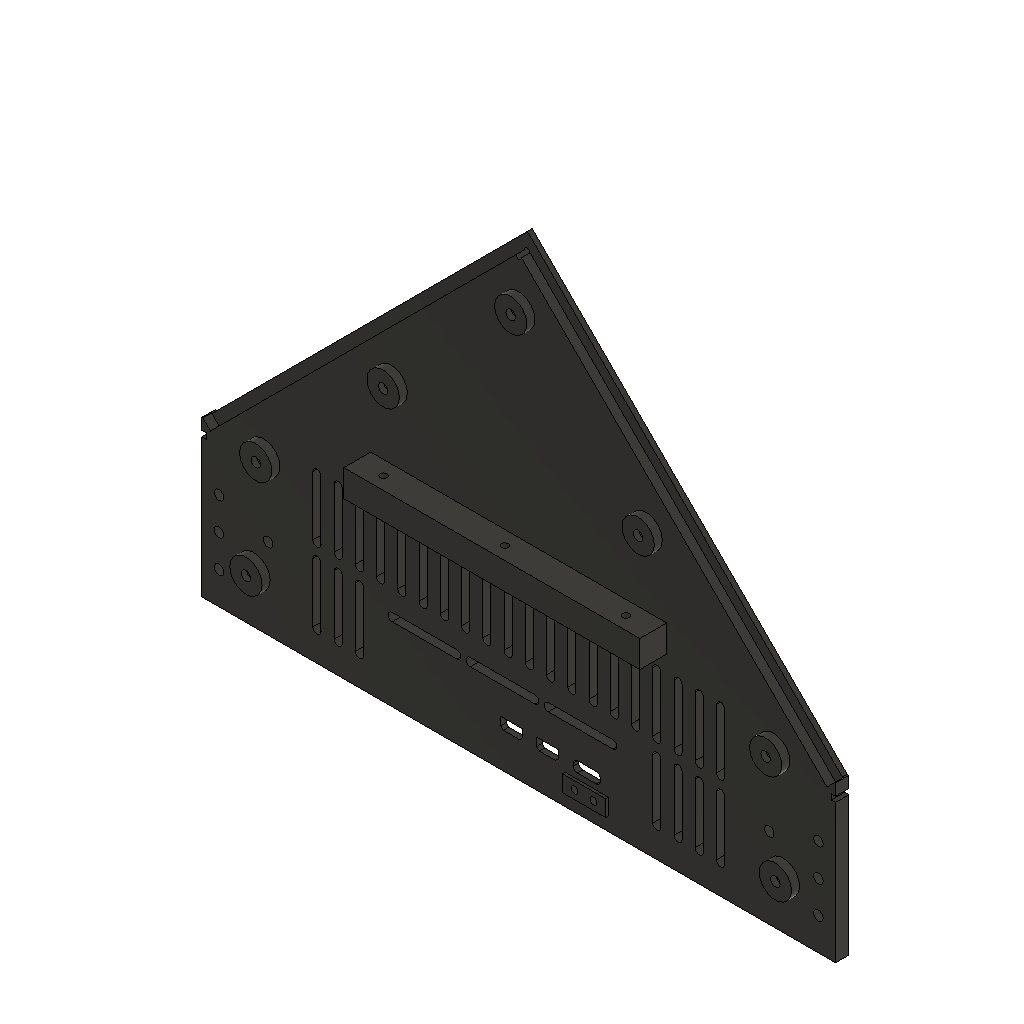
back (Autodesk Fusion 360 design; units mm, degrees)
Autodesk Fusion 360 part; units mm, degrees
sketch "Skizze1" plane through (0, 0, 0) normal (0, 1, 0) x (1, 0, 0)
  line L0 (-3.3486, -96.1672) -> (-1.6743, -99.0672)
  circle A0 centre (0, -113.552) radius 1
  line L1 (-1.6743, -99.0672) -> (1.6743, -99.0672)
  circle A1 centre (47.3762, -48.7911) radius 1.75
  circle A2 centre (47.3762, -48.7911) radius 6
  line L2 (116.137, 3.4146) -> (118.137, 3.4146)
  line L3 (96.4266, 1.4851) -> (98.1009, -1.4149)
  line L4 (93.078, -4.3149) -> (91.4037, -1.4149)
  line L5 (50.7248, -48.7911) -> (49.0505, -51.6911)
  line L6 (118.137, 3.4146) -> (118.137, 1.4146)
  line L7 (93.078, 1.4851) -> (96.4266, 1.4851)
  line L8 (1.6743, -99.0672) -> (3.3486, -96.1672)
  circle A3 centre (0, -96.1672) radius 1.75
  line L9 (114.552, 0) -> (117.3804, -2.8284)
  circle A4 centre (94.7523, -1.4149) radius 1.75
  line L10 (3.3486, -96.1672) -> (1.6743, -93.2672)
  circle A5 centre (94.7523, -1.4149) radius 6
  line L11 (0, -120.2089) -> (117.3804, -2.8284)
  line L12 (45.7018, -45.8911) -> (49.0505, -45.8911)
  circle A6 centre (-111.38, 31) radius 1.75
  line L13 (-49.0505, -45.8911) -> (-50.7248, -48.7911)
  line L14 (-45.7018, -45.8911) -> (-49.0505, -45.8911)
  line L15 (-100.0543, 34.1) -> (-96.7057, 34.1)
  circle A7 centre (-111.38, 43) radius 1.75
  line L16 (-118.137, -2.8284) -> (-118.137, 55)
  line L17 (-100.0543, 39.9) -> (-101.7286, 37)
  line L18 (-120.0068, 23.8396) -> (4.4419, -100.6092) construction
  circle A8 centre (-94.7523, -1.4149) radius 1.75
  line L19 (-14.6701, -110.8373) -> (106.0816, 9.9144) construction
  line L20 (-111.38, -4.6505) -> (-111.38, 58.1997) construction
  circle A9 centre (-98.38, 37) radius 6
  line L21 (-96.7057, 34.1) -> (-95.0314, 37)
  circle A10 centre (-94.7523, -1.4149) radius 6
  line L22 (-52.4459, 0) -> (345.6761, 0) construction
  line L23 (-118.137, 55) -> (118.137, 55)
  line L24 (-116.137, 1.4146) -> (-116.137, 3.4146)
  line L25 (-117.3804, -2.8284) -> (-118.137, -2.8284)
  line L26 (-114.552, 0) -> (0, -114.552)
  line L27 (-95.0314, 37) -> (-96.7057, 39.9)
  line L28 (-118.137, 3.4146) -> (-118.137, 1.4146)
  line L29 (-96.7057, 39.9) -> (-100.0543, 39.9)
  line L30 (-96.4266, 1.4851) -> (-98.1009, -1.4149)
  line L31 (-116.137, 3.4146) -> (-118.137, 3.4146)
  line L32 (-93.078, -4.3149) -> (-91.4037, -1.4149)
  line L33 (-91.4037, -1.4149) -> (-93.078, 1.4851)
  line L34 (-118.137, 1.4146) -> (-116.137, 1.4146)
  circle A11 centre (-93.137, 25) radius 1.75
  line L35 (-98.38, 29.5228) -> (-98.38, 65.4203) construction
  line L36 (-93.137, 11.8531) -> (-93.137, 59.4737) construction
  line L37 (-98.1009, -1.4149) -> (-96.4266, -4.3149)
  line L38 (-93.078, 1.4851) -> (-96.4266, 1.4851)
  circle A12 centre (-98.38, 37) radius 1.75
  line L39 (-96.4266, -4.3149) -> (-93.078, -4.3149)
  line L40 (-114.552, 0) -> (-117.3804, -2.8284)
  circle A13 centre (-111.38, 19) radius 1.75
  line L41 (-101.7286, 37) -> (-100.0543, 34.1)
  line L42 (91.4037, -1.4149) -> (93.078, 1.4851)
  circle A14 centre (-47.3762, -48.7911) radius 6
  line L43 (-44.0275, -48.7911) -> (-45.7018, -45.8911)
  line L44 (-45.7018, -51.6911) -> (-44.0275, -48.7911)
  line L45 (-49.0505, -51.6911) -> (-45.7018, -51.6911)
  circle A15 centre (-47.3762, -48.7911) radius 1.75
  line L46 (118.137, -2.8284) -> (118.137, 55)
  line L47 (100.0543, 34.1) -> (96.7057, 34.1)
  line L48 (-117.3804, -2.8284) -> (0, -120.2089)
  line L49 (96.7057, 39.9) -> (100.0543, 39.9)
  line L50 (100.0543, 39.9) -> (101.7286, 37)
  line L51 (0, -220.0498) -> (0, 135.0469) construction
  line L52 (111.38, -16.7918) -> (111.38, 73.2082) construction
  line L53 (-0.5511, 92.7863) -> (31.9162, 125.2536) construction
  circle A16 centre (111.38, 19) radius 1.75
  circle A17 centre (111.38, 43) radius 1.75
  line L54 (95.0314, 37) -> (96.7057, 39.9)
  circle A18 centre (111.38, 31) radius 1.75
  line L55 (-50.7248, -48.7911) -> (-49.0505, -51.6911)
  line L56 (116.137, 1.4146) -> (116.137, 3.4146)
  line L57 (101.7286, 37) -> (100.0543, 34.1)
  circle A19 centre (98.38, 37) radius 6
  circle A20 centre (93.137, 25) radius 1.75
  circle A21 centre (98.38, 37) radius 1.75
  line L58 (45.7018, -51.6911) -> (44.0275, -48.7911)
  line L59 (1.6743, -93.2672) -> (-1.6743, -93.2672)
  line L60 (118.137, 1.4146) -> (116.137, 1.4146)
  line L61 (96.7057, 34.1) -> (95.0314, 37)
  line L62 (98.1009, -1.4149) -> (96.4266, -4.3149)
  line L63 (49.0505, -45.8911) -> (50.7248, -48.7911)
  line L64 (-1.6743, -93.2672) -> (-3.3486, -96.1672)
  circle A22 centre (0, -96.1672) radius 6
  line L65 (44.0275, -48.7911) -> (45.7018, -45.8911)
  line L66 (49.0505, -51.6911) -> (45.7018, -51.6911)
  line L67 (96.4266, -4.3149) -> (93.078, -4.3149)
  line L68 (117.3804, -2.8284) -> (118.137, -2.8284)
  line L69 (0, -114.552) -> (114.552, 0)
  line L70 (34.8, 35.9) -> (-10.8, 35.9)
  line L71 (-10.8, 35.9) -> (-10.8, 43.9)
  line L72 (-10.8, 43.9) -> (34.8, 43.9)
  line L73 (34.8, 43.9) -> (34.8, 35.9)
  line L74 (37, 50) -> (-32, 50) construction
  line L75 (51.4459, 39.9) -> (-23, 39.9) construction
  line L76 (10.7, 28) -> (10.7, 48) construction
  line L77 (25.3, 21.2933) -> (25.3, 58) construction
  line L78 (-2.7, 28) -> (-2.7, 48) construction
  line L79 (21.8, 41.9) -> (28.8, 41.9)
  line L80 (30.3, 40.4) -> (30.3, 39.4)
  line L81 (28.8, 37.9) -> (21.8, 37.9)
  line L82 (20.3, 39.4) -> (20.3, 40.4)
  line L83 (20.3, 41.9) -> (30.3, 37.9) construction
  line L84 (30.3, 41.9) -> (20.3, 37.9) construction
  line L85 (7.7, 41.9) -> (13.7, 41.9)
  line L86 (14.7, 40.9) -> (14.7, 37.9)
  line L87 (14.7, 37.9) -> (6.7, 37.9)
  line L88 (6.7, 37.9) -> (6.7, 40.9)
  line L89 (6.7, 41.9) -> (14.7, 37.9) construction
  line L90 (14.7, 41.9) -> (6.7, 37.9) construction
  line L91 (-5.7, 41.9) -> (0.3, 41.9)
  line L92 (1.3, 40.9) -> (1.3, 37.9)
  line L93 (1.3, 37.9) -> (-6.7, 37.9)
  line L94 (-6.7, 37.9) -> (-6.7, 40.9)
  line L95 (-6.7, 41.9) -> (1.3, 37.9) construction
  line L96 (1.3, 41.9) -> (-6.7, 37.9) construction
  arc A23 (28.8, 37.9) -> (30.3, 39.4) centre (28.8, 39.4) ccw
  arc A24 (20.3, 39.4) -> (21.8, 37.9) centre (21.8, 39.4) ccw
  arc A25 (21.8, 41.9) -> (20.3, 40.4) centre (21.8, 40.4) ccw
  arc A26 (30.3, 40.4) -> (28.8, 41.9) centre (28.8, 40.4) ccw
  line L97 (1.3, 40.9) -> (0.3, 41.9)
  line L98 (-5.7, 41.9) -> (-6.7, 40.9)
  line L99 (7.7, 41.9) -> (6.7, 40.9)
  line L100 (13.7, 41.9) -> (14.7, 40.9)
  line L101 (38, 46.9) -> (16.3042, 46.9) construction
  line L102 (33.3, 43.9) -> (33.3, 50)
  line L103 (17.3, 43.9) -> (17.3, 50)
  line L104 (33.3, 50) -> (17.3, 50)
  line L105 (28.8, 44.4473) -> (28.8, 49) construction
  line L106 (21.8, 44.3848) -> (21.8, 49.4152) construction
  circle A27 centre (28.8, 46.9) radius 1.25
  circle A28 centre (21.8, 46.9) radius 1.25
  line L107 (27.5298, 49.1) -> (26.2597, 46.9)
  line L108 (26.2597, 46.9) -> (27.5298, 44.7)
  line L109 (27.5298, 44.7) -> (30.0702, 44.7)
  line L110 (30.0702, 44.7) -> (31.3403, 46.9)
  line L111 (31.3403, 46.9) -> (30.0702, 49.1)
  line L112 (30.0702, 49.1) -> (27.5298, 49.1)
  line L113 (20.5298, 49.1) -> (19.2597, 46.9)
  line L114 (19.2597, 46.9) -> (20.5298, 44.7)
  line L115 (20.5298, 44.7) -> (23.0702, 44.7)
  line L116 (23.0702, 44.7) -> (24.3403, 46.9)
  line L117 (24.3403, 46.9) -> (23.0702, 49.1)
  line L118 (23.0702, 49.1) -> (20.5298, 49.1)
  line L119 (130, -23) -> (-128.9642, -23) construction
  line L120 (-55, -13) -> (55, -13)
  line L121 (55, -13) -> (55, -23)
  line L122 (55, -23) -> (-55, -23)
  line L123 (-55, -23) -> (-55, -13)
  line L124 (-55, -13) -> (55, -23) construction
  line L125 (55, -13) -> (-55, -23) construction
  line L126 (65.5233, 43.1) -> (-51.9095, 43.1) construction
  line L127 (67.4251, 23.1) -> (-80, 23.1) construction
  line L128 (73.5779, 26.1) -> (-77.6362, 26.1) construction
  line L129 (36.5, 19) -> (36.5, 58) construction
  line L130 (-48.5, 15) -> (-48.5, 73) construction
  line L131 (-47, 27.6) -> (-23, 27.6)
  line L132 (-23, 27.6) -> (-23, 24.6) construction
  line L133 (-23, 24.6) -> (-47, 24.6)
  line L134 (-47, 24.6) -> (-47, 27.6) construction
  line L135 (-47, 27.6) -> (-23, 24.6) construction
  line L136 (-23, 27.6) -> (-47, 24.6) construction
  line L137 (-18, 27.6) -> (6, 27.6)
  line L138 (6, 27.6) -> (6, 24.6) construction
  line L139 (6, 24.6) -> (-18, 24.6)
  line L140 (-18, 24.6) -> (-18, 27.6) construction
  line L141 (-18, 27.6) -> (6, 24.6) construction
  line L142 (6, 27.6) -> (-18, 24.6) construction
  line L143 (11, 27.6) -> (35, 27.6)
  line L144 (35, 27.6) -> (35, 24.6) construction
  line L145 (35, 24.6) -> (11, 24.6)
  line L146 (11, 24.6) -> (11, 27.6) construction
  line L147 (11, 27.6) -> (35, 24.6) construction
  line L148 (35, 27.6) -> (11, 24.6) construction
  arc A29 (-47, 27.6) -> (-47, 24.6) centre (-47, 26.1) ccw
  arc A30 (-23, 24.6) -> (-23, 27.6) centre (-23, 26.1) ccw
  arc A31 (-18, 27.6) -> (-18, 24.6) centre (-18, 26.1) ccw
  arc A32 (6, 24.6) -> (6, 27.6) centre (6, 26.1) ccw
  arc A33 (11.4382, 27.5346) -> (11, 24.6) centre (11, 26.1) ccw
  arc A34 (35, 24.6) -> (35, 27.6) centre (35, 26.1) ccw
  line L149 (84.4109, 5) -> (-85.7418, 5) construction
  line L150 (73.5, 16) -> (76.5, 16) construction
  line L151 (76.5, 16) -> (76.5, -6)
  line L152 (76.5, -6) -> (73.5, -6) construction
  line L153 (73.5, -6) -> (73.5, 16)
  line L154 (73.5, 16) -> (76.5, -6) construction
  line L155 (76.5, 16) -> (73.5, -6) construction
  arc A35 (73.5, -6) -> (76.5, -6) centre (75, -6) ccw
  arc A36 (76.5, 16) -> (73.5, 16) centre (75, 16) ccw
  line L156 (65.6053, -6) -> (65.6053, 16)
  arc A37 (65.6053, -6) -> (68.6053, -6) centre (67.1053, -6) ccw
  line L157 (68.6053, 16) -> (68.6053, -6)
  arc A38 (68.6053, 16) -> (65.6053, 16) centre (67.1053, 16) ccw
  line L158 (57.7105, -6) -> (57.7105, 16)
  arc A39 (57.7105, -6) -> (60.7105, -6) centre (59.2105, -6) ccw
  line L159 (60.7105, 16) -> (60.7105, -6)
  arc A40 (60.7105, 16) -> (57.7105, 16) centre (59.2105, 16) ccw
  line L160 (49.8158, -6) -> (49.8158, 16)
  arc A41 (49.8158, -6) -> (52.8158, -6) centre (51.3158, -6) ccw
  line L161 (52.8158, 16) -> (52.8158, -6)
  arc A42 (52.8158, 16) -> (49.8158, 16) centre (51.3158, 16) ccw
  line L162 (41.9211, -6) -> (41.9211, 16)
  arc A43 (41.9211, -6) -> (44.9211, -6) centre (43.4211, -6) ccw
  line L163 (44.9211, 16) -> (44.9211, -6)
  arc A44 (44.9211, 16) -> (41.9211, 16) centre (43.4211, 16) ccw
  line L164 (34.0263, -6) -> (34.0263, 16)
  arc A45 (34.0263, -6) -> (37.0263, -6) centre (35.5263, -6) ccw
  line L165 (37.0263, 16) -> (37.0263, -6)
  arc A46 (37.0263, 16) -> (34.0263, 16) centre (35.5263, 16) ccw
  line L166 (26.1316, -6) -> (26.1316, 16)
  arc A47 (26.1316, -6) -> (29.1316, -6) centre (27.6316, -6) ccw
  line L167 (29.1316, 16) -> (29.1316, -6)
  arc A48 (29.1316, 16) -> (26.1316, 16) centre (27.6316, 16) ccw
  line L168 (18.2368, -6) -> (18.2368, 16)
  arc A49 (18.2368, -6) -> (21.2368, -6) centre (19.7368, -6) ccw
  line L169 (21.2368, 16) -> (21.2368, -6)
  arc A50 (21.2368, 16) -> (18.2368, 16) centre (19.7368, 16) ccw
  line L170 (10.3421, -6) -> (10.3421, 16)
  arc A51 (10.3421, -6) -> (13.3421, -6) centre (11.8421, -6) ccw
  line L171 (13.3421, 16) -> (13.3421, -6)
  arc A52 (13.3421, 16) -> (10.3421, 16) centre (11.8421, 16) ccw
  line L172 (2.4474, -6) -> (2.4474, 16)
  arc A53 (2.4474, -6) -> (5.4474, -6) centre (3.9474, -6) ccw
  line L173 (5.4474, 16) -> (5.4474, -6)
  arc A54 (5.4474, 16) -> (2.4474, 16) centre (3.9474, 16) ccw
  line L174 (-5.4474, -6) -> (-5.4474, 16)
  arc A55 (-5.4474, -6) -> (-2.4474, -6) centre (-3.9474, -6) ccw
  line L175 (-2.4474, 16) -> (-2.4474, -6)
  arc A56 (-2.4474, 16) -> (-5.4474, 16) centre (-3.9474, 16) ccw
  line L176 (-13.3421, -6) -> (-13.3421, 16)
  arc A57 (-13.3421, -6) -> (-10.3421, -6) centre (-11.8421, -6) ccw
  line L177 (-10.3421, 16) -> (-10.3421, -6)
  arc A58 (-10.3421, 16) -> (-13.3421, 16) centre (-11.8421, 16) ccw
  line L178 (-21.2368, -6) -> (-21.2368, 16)
  arc A59 (-21.2368, -6) -> (-18.2368, -6) centre (-19.7368, -6) ccw
  line L179 (-18.2368, 16) -> (-18.2368, -6)
  arc A60 (-18.2368, 16) -> (-21.2368, 16) centre (-19.7368, 16) ccw
  line L180 (-29.1316, -6) -> (-29.1316, 16)
  arc A61 (-29.1316, -6) -> (-26.1316, -6) centre (-27.6316, -6) ccw
  line L181 (-26.1316, 16) -> (-26.1316, -6)
  arc A62 (-26.1316, 16) -> (-29.1316, 16) centre (-27.6316, 16) ccw
  line L182 (-37.0263, -6) -> (-37.0263, 16)
  arc A63 (-37.0263, -6) -> (-34.0263, -6) centre (-35.5263, -6) ccw
  line L183 (-34.0263, 16) -> (-34.0263, -6)
  arc A64 (-34.0263, 16) -> (-37.0263, 16) centre (-35.5263, 16) ccw
  line L184 (-44.9211, -6) -> (-44.9211, 16)
  arc A65 (-44.9211, -6) -> (-41.9211, -6) centre (-43.4211, -6) ccw
  line L185 (-41.9211, 16) -> (-41.9211, -6)
  arc A66 (-41.9211, 16) -> (-44.9211, 16) centre (-43.4211, 16) ccw
  line L186 (-52.8158, -6) -> (-52.8158, 16)
  arc A67 (-52.8158, -6) -> (-49.8158, -6) centre (-51.3158, -6) ccw
  line L187 (-49.8158, 16) -> (-49.8158, -6)
  arc A68 (-49.8158, 16) -> (-52.8158, 16) centre (-51.3158, 16) ccw
  line L188 (-60.7105, -6) -> (-60.7105, 16)
  arc A69 (-60.7105, -6) -> (-57.7105, -6) centre (-59.2105, -6) ccw
  line L189 (-57.7105, 16) -> (-57.7105, -6)
  arc A70 (-57.7105, 16) -> (-60.7105, 16) centre (-59.2105, 16) ccw
  line L190 (-68.6053, -6) -> (-68.6053, 16)
  arc A71 (-68.6053, -6) -> (-65.6053, -6) centre (-67.1053, -6) ccw
  line L191 (-65.6053, 16) -> (-65.6053, -6)
  arc A72 (-65.6053, 16) -> (-68.6053, 16) centre (-67.1053, 16) ccw
  line L192 (-76.5, -6) -> (-76.5, 16)
  arc A73 (-76.5, -6) -> (-73.5, -6) centre (-75, -6) ccw
  line L193 (-73.5, 16) -> (-73.5, -6)
  arc A74 (-73.5, 16) -> (-76.5, 16) centre (-75, 16) ccw
  line L194 (86.8847, 33) -> (-89.6414, 33) construction
  line L195 (73.5, 44) -> (76.5, 44) construction
  line L196 (76.5, 44) -> (76.5, 22)
  line L197 (76.5, 22) -> (73.5, 22) construction
  line L198 (73.5, 22) -> (73.5, 44)
  line L199 (73.5, 44) -> (76.5, 22) construction
  line L200 (76.5, 44) -> (73.5, 22) construction
  arc A75 (73.5, 22) -> (76.5, 22) centre (75, 22) ccw
  arc A76 (76.5, 44) -> (73.5, 44) centre (75, 44) ccw
  line L201 (65.605, 22) -> (65.605, 44)
  arc A77 (65.605, 22) -> (68.605, 22) centre (67.105, 22) ccw
  line L202 (68.605, 44) -> (68.605, 22)
  arc A78 (68.605, 44) -> (65.605, 44) centre (67.105, 44) ccw
  line L203 (57.71, 22) -> (57.71, 44)
  arc A79 (57.71, 22) -> (60.71, 22) centre (59.21, 22) ccw
  line L204 (60.71, 44) -> (60.71, 22)
  arc A80 (60.71, 44) -> (57.71, 44) centre (59.21, 44) ccw
  line L205 (49.815, 22) -> (49.815, 44)
  arc A81 (49.815, 22) -> (52.815, 22) centre (51.315, 22) ccw
  line L206 (52.815, 44) -> (52.815, 22)
  arc A82 (52.815, 44) -> (49.815, 44) centre (51.315, 44) ccw
  line L207 (-76.5, 44) -> (-73.5, 44) construction
  line L208 (-73.5, 44) -> (-73.5, 22)
  line L209 (-73.5, 22) -> (-76.5, 22) construction
  line L210 (-76.5, 22) -> (-76.5, 44)
  line L211 (-76.5, 44) -> (-73.5, 22) construction
  line L212 (-73.5, 44) -> (-76.5, 22) construction
  arc A83 (-73.5, 22.0002) -> (-73.5, 22) centre (-72.7991, 22) ccw
  arc A84 (-73.5, 44) -> (-76.5, 44) centre (-75, 44) ccw
  arc A85 (-76.5, 22) -> (-73.5, 22.0002) centre (-75, 22) ccw
  line L213 (-68.605, 22) -> (-68.605, 44)
  arc A86 (-68.605, 22) -> (-65.605, 22.0002) centre (-67.105, 22) ccw
  line L214 (-65.605, 44) -> (-65.605, 22)
  arc A87 (-65.605, 44) -> (-68.605, 44) centre (-67.105, 44) ccw
  line L215 (-60.71, 22) -> (-60.71, 44)
  arc A88 (-60.71, 22) -> (-57.71, 22.0002) centre (-59.21, 22) ccw
  line L216 (-57.71, 44) -> (-57.71, 22)
  arc A89 (-57.71, 44) -> (-60.71, 44) centre (-59.21, 44) ccw
  point P0 (114.552, 0)
  point P1 (-114.552, 0)
  point P2 (-94.7523, -1.4149)
  point P3 (-98.38, 37)
  point P4 (0, -96.1672)
  point P5 (0, -16.1)
  point P6 (0, 46.6)
  point P7 (-47.3762, -48.7911)
  point P8 (25.3, 39.9)
  point P9 (10.7, 39.9)
  point P10 (-2.7, 39.9)
  point P11 (28.8, 46.9)
  point P12 (21.8, 46.9)
  point P13 (0, -18)
  point P14 (-35, 26.1)
  point P15 (-6, 26.1)
  point P16 (23, 26.1)
  point P17 (75, 5)
  point P18 (75, 33)
  point P19 (75, 22)
  point P20 (-75, 33)
  dimension "d1" = 55
  dimension "d2" = 45
  dimension "d3" = 4
  dimension "d4" = 4
  dimension "d5" = 12
  dimension "d6" = 12
  dimension "d7" = 12
  dimension "d8" = 3.5
  dimension "d9" = 3.5
  dimension "d10" = 3.5
  dimension "d11" = 12
  dimension "d12" = 12
  dimension "d13" = 12
  dimension "d14" = 3.5
  dimension "d15" = 3.5
  dimension "d16" = 3.5
  dimension "d17" = 18
  dimension "d18" = 12
  dimension "d19" = 3.5
  dimension "d20" = 5.8
  dimension "d21" = 3.5
  dimension "d22" = 30
  dimension "d23" = 13
  dimension "d25" = 13
  dimension "d26" = 3.5
  dimension "d27" = 12
  dimension "d28" = 5.8
  dimension "d29" = 12
  dimension "d30" = 3.5
  dimension "d31" = 5.8
  dimension "d33" = 12
  dimension "d34" = 3.5
  dimension "d35" = 5.8
  dimension "d42" = 118.137
  dimension "d43" = 6.757
  dimension "d44" = 19.757
  dimension "d45" = 25
  dimension "d46" = 3.585
  dimension "d47" = 118.137
  dimension "d48" = 6.757
  dimension "d49" = 3.585
  dimension "d50" = 4.243
  dimension "d51" = 2
  dimension "d52" = 2
  dimension "d53" = 2
  dimension "d54" = 11.1
  dimension "d55" = 5
  dimension "d56" = 34.8
  dimension "d57" = 10.8
  dimension "d58" = 4
  dimension "d59" = 4
  dimension "d60" = 21.5
  dimension "d61" = 14.6
  dimension "d62" = 13.4
  dimension "d63" = 4
  dimension "d64" = 10
  dimension "d65" = 1.5
  dimension "d66" = 4
  dimension "d67" = 8
  dimension "d68" = 4
  dimension "d69" = 8
  dimension "d70" = 1
  dimension "d71" = 1
  dimension "d72" = 1
  dimension "d73" = 1
  dimension "d74" = 1
  dimension "d75" = 1
  dimension "d76" = 1
  dimension "d77" = 1
  dimension "d78" = 7
  dimension "d79" = 8
  dimension "d80" = 8
  dimension "d81" = 3.5
  dimension "d82" = 3.5
  dimension "d83" = 2.5
  dimension "d84" = 2.5
  dimension "d85" = 4.4
  dimension "d86" = 4.4
  dimension "d91" = 67
  dimension "d92" = 67
  dimension "d113" = 78
  dimension "d114" = 10
  dimension "d115" = 110
  dimension "d133" = 3.2
  dimension "d134" = 20
  dimension "d135" = 3
  dimension "d136" = 11.2
  dimension "d137" = 85
  dimension "d138" = 3
  dimension "d139" = 3
  dimension "d140" = 3
  dimension "d141" = 24
  dimension "d142" = 24
  dimension "d143" = 42.5
  dimension "d144" = 24
  dimension "d145" = 29
  dimension "d146" = 29
  dimension "d147" = 3
  dimension "d148" = 22
  dimension "d151" = -150
  dimension "d152" = 0
  dimension "d153" = 75
  dimension "d154" = 50
  dimension "d155" = 3
  dimension "d156" = 22
  dimension "d158" = 75
  dimension "d159" = 22
  dimension "d162" = -23.685
  dimension "d163" = 0
  dimension "d164" = 3
  dimension "d165" = 22
  dimension "d166" = 75
  dimension "d169" = 15.79
  dimension "d170" = 0
  constraint horizontal L22
  constraint coincident origin L51
  constraint coincident origin L22
  constraint horizontal L23
  constraint coincident P1 L22
  constraint coincident P0 L22
  constraint coincident P1 L26.start
  constraint coincident L26.end L51
  constraint coincident P0 L9.start
  constraint perpendicular L26 L40
  constraint perpendicular L9 L69
  constraint horizontal L68
  constraint perpendicular L20 L23
  constraint perpendicular L23 L52
  constraint coincident A17.centre L52
  constraint coincident A18.centre L52
  constraint coincident A16.centre L52
  constraint coincident A7.centre L20
  constraint coincident A6.centre L20
  constraint coincident A13.centre L20
  constraint perpendicular L23 L35
  constraint coincident P3 L35
  constraint concentric A9 A12
  constraint coincident P3 A9.centre
  constraint horizontal L29
  constraint perpendicular L23 L36
  constraint coincident A11.centre L36
  constraint parallel L18 L26
  constraint parallel L19 L69
  constraint coincident P4 L51
  constraint coincident P4 L18
  constraint concentric A3 A22
  constraint coincident P4 A3.centre
  constraint horizontal L1
  constraint coincident P7 L18
  constraint concentric A14 A15
  constraint coincident P7 A14.centre
  constraint horizontal L14
  constraint perpendicular L18 L53
  constraint coincident P2 L18
  constraint coincident P2 L53
  constraint concentric A8 A10
  constraint coincident P2 A8.centre
  constraint horizontal L38
  constraint symmetric A9 L51 A19
  constraint symmetric A12 L51 A21
  constraint symmetric L17.start L49.end L51
  constraint symmetric L17.end L50.end L51
  constraint symmetric L15.start L47.start L51
  constraint symmetric L15.end L47.end L51
  constraint symmetric L54.start L21.end L51
  constraint symmetric L49.start L27.end L51
  constraint symmetric A11 L51 A20
  constraint symmetric A1 A15 L51
  constraint symmetric A2 A14 L51
  constraint symmetric L12.end L13.start L51
  constraint symmetric L13.end L5.start L51
  constraint symmetric L5.end L45.start L51
  constraint symmetric L58.start L44.start L51
  constraint symmetric L58.end L43.start L51
  constraint symmetric L12.start L14.start L51
  constraint symmetric A4 A8 L51
  constraint symmetric A5 A10 L51
  constraint symmetric L3.start L30.start L51
  constraint symmetric L3.end L30.end L51
  constraint symmetric L37.end L62.end L51
  constraint symmetric L32.start L4.start L51
  constraint symmetric L32.end L4.end L51
  constraint symmetric L33.end L7.start L51
  constraint coincident P6 L51
  constraint coincident P5 L51
  constraint coincident L11.start L51
  constraint parallel L26 L48
  constraint coincident L16.end L23
  constraint perpendicular L16 L23
  constraint coincident L25.end L16
  constraint coincident L16.end L23.start
  constraint coincident L46.start L68
  constraint coincident L46.end L23
  constraint perpendicular L23 L46
  constraint coincident L23.end L46.end
  constraint coincident L46.start L68.end
  constraint horizontal L34
  constraint vertical L24
  constraint horizontal L31
  constraint vertical L28
  constraint coincident L28.end L16
  constraint symmetric L28.end L6.end L51
  constraint symmetric L24.start L56.start L51
  constraint symmetric L24.end L2.start L51
  constraint symmetric L28.start L2.end L51
  constraint coincident A0.centre L51
  constraint coincident L26.end A0
  constraint horizontal L70
  constraint vertical L71
  constraint horizontal L72
  constraint vertical L73
  constraint perpendicular L71 L74
  constraint perpendicular L51 L75
  constraint perpendicular L72 L76
  constraint perpendicular L72 L77
  constraint perpendicular L72 L78
  constraint horizontal L79
  constraint perpendicular L79 L80
  constraint parallel L79 L81
  constraint parallel L80 L82
  constraint coincident L83 P8
  constraint coincident L84 P8
  constraint coincident L77 P8
  constraint coincident L75 P8
  constraint horizontal L85
  constraint perpendicular L85 L86
  constraint parallel L85 L87
  constraint parallel L86 L88
  constraint coincident L89 P9
  constraint coincident L90 P9
  constraint coincident L75 P9
  constraint coincident L76 P9
  constraint horizontal L91
  constraint perpendicular L91 L92
  constraint parallel L91 L93
  constraint parallel L92 L94
  constraint coincident L95 P10
  constraint coincident L96 P10
  constraint coincident L78 P10
  constraint coincident L75 P10
  constraint coincident L83.end L81
  constraint coincident L83.end L80
  constraint tangent L81 A23
  constraint tangent L80 A23
  constraint coincident L84.end L81
  constraint coincident L84.end L82
  constraint tangent L81 A24
  constraint tangent L82 A24
  constraint equal A23 A24
  constraint coincident L83.start L82
  constraint coincident L83.start L79
  constraint tangent L82 A25
  constraint tangent L79 A25
  constraint equal A23 A25
  constraint coincident L84.start L79
  constraint coincident L84.start L80
  constraint tangent L79 A26
  constraint tangent L80 A26
  constraint equal A23 A26
  constraint coincident L96.start L92
  constraint coincident L96.start L91
  constraint coincident L95.start L91
  constraint coincident L95.start L94
  constraint coincident L89.start L85
  constraint coincident L89.start L88
  constraint coincident L90.start L85
  constraint coincident L90.start L86
  constraint perpendicular L77 L101
  constraint coincident L72 L102.start
  constraint coincident L74 L102.end
  constraint perpendicular L74 L102
  constraint coincident L72 L103.start
  constraint coincident L74 L103.end
  constraint perpendicular L74 L103
  constraint perpendicular L101 L105
  constraint perpendicular L101 L106
  constraint coincident L105 P11
  constraint coincident L101 P11
  constraint midpoint L106 P12
  constraint coincident L101 P12
  constraint coincident P11 A27.centre
  constraint coincident P12 A28.centre
  constraint horizontal L118
  constraint horizontal L112
  constraint coincident P4 L19
  constraint horizontal L25
  constraint horizontal L119
  constraint horizontal L120
  constraint perpendicular L120 L121
  constraint parallel L120 L122
  constraint parallel L121 L123
  constraint coincident L124 P13
  constraint coincident L125 P13
  constraint coincident L51 P13
  constraint coincident L119 L122.end
  constraint horizontal L126
  constraint perpendicular L51 L127
  constraint horizontal L128
  constraint perpendicular L23 L129
  constraint perpendicular L127 L130
  constraint horizontal L131
  constraint perpendicular L131 L132
  constraint parallel L131 L133
  constraint parallel L132 L134
  constraint coincident L135 P14
  constraint coincident L136 P14
  constraint coincident L128 P14
  constraint horizontal L137
  constraint perpendicular L137 L138
  constraint parallel L137 L139
  constraint parallel L138 L140
  constraint coincident L141 P15
  constraint coincident L142 P15
  constraint coincident L128 P15
  constraint horizontal L143
  constraint perpendicular L143 L144
  constraint parallel L143 L145
  constraint parallel L144 L146
  constraint coincident L147 P16
  constraint coincident L148 P16
  constraint coincident L128 P16
  constraint midpoint L134 A29.centre
  constraint midpoint L132 A30.centre
  constraint midpoint L140 A31.centre
  constraint midpoint L138 A32.centre
  constraint midpoint L146 A33.centre
  constraint midpoint L144 A34.centre
  constraint perpendicular L129 L149
  constraint horizontal L150
  constraint perpendicular L150 L151
  constraint parallel L150 L152
  constraint parallel L151 L153
  constraint coincident L154 P17
  constraint coincident L155 P17
  constraint coincident L149 P17
  constraint coincident L152 A35.centre
  constraint coincident L150 A36.centre
  constraint coincident L150.start L153.end
  constraint coincident L152.end L153.start
  constraint perpendicular L78 L194
  constraint horizontal L195
  constraint perpendicular L195 L196
  constraint parallel L195 L197
  constraint parallel L196 L198
  constraint coincident L199 P18
  constraint coincident L200 P18
  constraint coincident L194 P18
  constraint midpoint L197 P19
  constraint coincident L197 L198.start
  constraint coincident L197 P19
  constraint coincident L195 L198.end
  constraint coincident L195 A76.centre
  constraint coincident L195.start L198.end
  constraint coincident L197.end L198.start
  constraint horizontal L207
  constraint perpendicular L207 L208
  constraint parallel L207 L209
  constraint parallel L208 L210
  constraint coincident L211 P20
  constraint coincident L212 P20
  constraint coincident L194 P20
  constraint coincident L209 A83.centre
  constraint coincident L207 A84.centre
  constraint coincident L207.start L210.end
  constraint coincident L209 A85.centre
  constraint coincident L209.end L210.start
  measures "d1" distance of L22 L23
  measures "d2" angle of L51 L69
  measures "d3" distance of P1 L25.start
  measures "d4" distance of P0 L9.end
  measures "d5" distance of A16.centre A18.centre
  measures "d6" distance of A18.centre A17.centre
  measures "d7" distance of A17.centre L23
  measures "d8" diameter of A17
  measures "d9" diameter of A18
  measures "d10" diameter of A16
  measures "d11" distance of A13.centre A6.centre
  measures "d12" distance of A7.centre A6.centre
  measures "d13" distance of A7.centre L23
  measures "d14" diameter of A13
  measures "d15" diameter of A6
  measures "d16" diameter of A7
  measures "d17" distance of P3 L23
  measures "d18" diameter of A9
  measures "d19" diameter of A12
  measures "d20" distance of L15 L29
  measures "d21" diameter of A11
  measures "d22" distance of A11.centre L23
  measures "d23" distance of L18 L26
  measures "d25" distance of L19 L69
  measures "d26" diameter of A3
  measures "d27" diameter of A22
  measures "d28" distance of L1 L59
  measures "d29" diameter of A14
  measures "d30" diameter of A15
  measures "d31" distance of L14 L45
  measures "d33" diameter of A10
  measures "d34" diameter of A8
  measures "d35" distance of L38 L39
  measures "d42" distance of L16 L51
  measures "d43" distance of L16 L20
  measures "d44" distance of L16 L35
  measures "d45" distance of L16 L36
  measures "d46" distance of P1 L16
  measures "d47" distance of L46 L51
  measures "d48" distance of L46 L52
  measures "d49" distance of P0 L46
  measures "d50" distance of L16.start L34
  measures "d51" distance of L16 L24
  measures "d52" distance of L31 L34
  measures "d53" diameter of A0
  measures "d54" distance of L23 L72
  measures "d55" distance of L23 L74
  measures "d56" distance of L51 L73
  measures "d57" distance of L51 L71
  measures "d58" distance of L72 L75
  measures "d59" distance of L70 L75
  measures "d60" distance of L71 L76
  measures "d61" distance of L76 L77
  measures "d62" distance of L76 L78
  measures "d63" distance of L79 L81
  measures "d64" distance of L80 L82
  measures "d65" radius of A23
  measures "d66" distance of L85 L87
  measures "d67" distance of L86 L88
  measures "d68" distance of L91 L93
  measures "d69" distance of L92 L94
  measures "d70" distance of L96.start L92.start
  measures "d71" distance of L96.start L91.end
  measures "d72" distance of L95.start L91.start
  measures "d73" distance of L95.start L94.end
  measures "d74" distance of L89.start L85.start
  measures "d75" distance of L89.start L88.end
  measures "d76" distance of L90.start L85.end
  measures "d77" distance of L90.start L86.start
  measures "d78" distance of L75 L101
  measures "d79" distance of L77 L103
  measures "d80" distance of L77 L102
  measures "d81" distance of L77 L106
  measures "d82" distance of L77 L105
  measures "d83" diameter of A28
  measures "d84" diameter of A27
  measures "d85" distance of L115 L118
  measures "d86" distance of L109 L112
  measures "d91" distance of P4 P7
  measures "d92" distance of P7 P2
  measures "d113" distance of L23 L119
  measures "d114" distance of L120 L122
  measures "d115" distance of L121 L123
  measures "d133" distance of L75 L126
  measures "d134" distance of L126 L127
  measures "d135" distance of L127 L128
  measures "d136" distance of L77 L129
  measures "d137" distance of L129 L130
  measures "d138" distance of L143 L145
  measures "d139" distance of L137 L139
  measures "d140" distance of L131 L133
  measures "d141" distance of L132 L134
  measures "d142" distance of L138 L140
  measures "d143" distance of L129 P15
  measures "d144" distance of L144 L146
  measures "d145" distance of P14 P15
  measures "d146" distance of P15 P16
  measures "d147" distance of L151 L153
  measures "d148" distance of L150 L152
  measures "d153" distance of L51 P17
  measures "d154" distance of L23 L149
  measures "d155" distance of L196 L198
  measures "d156" distance of L195 P19
  measures "d158" distance of L51 P18
  measures "d159" distance of L23 L194
  measures "d164" distance of L208 L210
  measures "d165" distance of L207 L209
  measures "d166" distance of L51 P20
extrude "Extrusion1" add sketch "Skizze1" along normal blind 2 contours L0 L1 L8 L10 L59 L64 | A0 L9 L11 L26 L40 L48 L69 | A0 L2 L9 L16 L23 L24 L25 L26 L31 L34 L40 L46 L56 L60 L68 L69 | A1 | A2 | L3 L4 L7 L42 L62 L67 | L5 L12 L58 L63 L65 L66 | A3 | A4 | A5 | A6 | L13 L14 L43 L44 L45 L55 | L15 L17 L21 L27 L29 L41 | A7 | A8 | A9 | A10 | L30 L32 L33 L37 L38 L39 | A11 | A12 | A13 | A14 | A15 | L47 L49 L50 L54 L57 L61 | A16 | A17 | A18 | A19 | A20 | A21 | A22 | L70 L71 L72 L73 | L72 L102 L103 L104 | L79 L80 L81 L82 A23 A24 A25 A26 | L85 L86 L87 L88 L99 L100 | L91 L92 L93 L94 L97 L98 | A27 | A28 | L107 L108 L109 L110 L111 L112 | L113 L114 L115 L116 L117 L118 | L120 L121 L122 L123 | A83
extrude "Extrusion2" add sketch "Skizze1" against normal blind 3 contours L0 L1 L8 L10 L59 L64 | A0 L2 L9 L16 L23 L24 L25 L26 L31 L34 L40 L46 L56 L60 L68 L69 | A1 | A2 | L3 L4 L7 L42 L62 L67 | L5 L12 L58 L63 L65 L66 | A3 | A4 | A5 | A6 | L13 L14 L43 L44 L45 L55 | L15 L17 L21 L27 L29 L41 | A7 | A8 | A9 | A10 | L30 L32 L33 L37 L38 L39 | A11 | A12 | A13 | A14 | A15 | L47 L49 L50 L54 L57 L61 | A16 | A17 | A18 | A19 | A20 | A21 | A22 | L70 L71 L72 L73 | L72 L102 L103 L104 | L79 L80 L81 L82 A23 A24 A25 A26 | L85 L86 L87 L88 L99 L100 | L91 L92 L93 L94 L97 L98 | A27 | A28 | L107 L108 L109 L110 L111 L112 | L113 L114 L115 L116 L117 L118 | L120 L121 L122 L123 | A83
extrude "Extrusion3" add sketch "Skizze1" against normal blind 6 contours L0 L1 L8 L10 L59 L64 | A2 | L3 L4 L7 L42 L62 L67 | L5 L12 L58 L63 L65 L66 | A5 | L13 L14 L43 L44 L45 L55 | L15 L17 L21 L27 L29 L41 | A9 | A10 | L30 L32 L33 L37 L38 L39 | A14 | L47 L49 L50 L54 L57 L61 | A19 | A22
extrude "Extrusion4" cut sketch "Skizze1" along normal mid plane 6 contours A1 | A3 | A4 | A6 | A7 | A8 | A11 | A12 | A13 | A15 | A16 | A17 | A18 | A20 | A21 | L79 L80 L81 L82 A23 A24 A25 A26 | L85 L86 L87 L88 L99 L100 | L91 L92 L93 L94 L97 L98 | A27 | A28
extrude "Extrusion5" cut sketch "Skizze1" against normal blind 4 contours L0 L1 L8 L10 L59 L64 | L3 L4 L7 L42 L62 L67 | L5 L12 L58 L63 L65 L66 | L13 L14 L43 L44 L45 L55 | L15 L17 L21 L27 L29 L41 | L30 L32 L33 L37 L38 L39 | L47 L49 L50 L54 L57 L61
extrude "Extrusion6" add sketch "Skizze1" against normal blind 1.3 contours L0 L1 L8 L10 L59 L64 | L3 L4 L7 L42 L62 L67 | L5 L12 L58 L63 L65 L66 | L13 L14 L43 L44 L45 L55 | L15 L17 L21 L27 L29 L41 | L30 L32 L33 L37 L38 L39 | L47 L49 L50 L54 L57 L61
extrude "Extrusion7" cut sketch "Skizze1" along normal blind 2 and the other way blind 1 contours L70 L71 L72 L73
chamfer "Fase1" distance 1 angle 45 4 edges at (12, 2, -43.9) (12, 2, -35.9) (-10.8, 2, -39.9) (34.8, 2, -39.9) tangent chain off
extrude "Extrusion8" add sketch "Skizze1" against normal blind 4 contours L72 L102 L103 L104 | L107 L108 L109 L110 L111 L112 | L113 L114 L115 L116 L117 L118
extrude "Extrusion9" cut sketch "Skizze1" against normal blind 1.8 contours L107 L108 L109 L110 L111 L112 | L113 L114 L115 L116 L117 L118
move_face "Flächen versetzen1" offset -0.2 4 faces at (-118.137, 0.3333, -37.8049) (-118.137, 0.3333, -0.0002) (118.137, 0.3333, -37.8049) (118.137, 0.3333, -0.0002)
move_face "Flächen versetzen2" offset -0.2 6 faces at (117.937, 0.3333, -37.8049) (117.937, 0.3333, -0.0002) (39.1268, 1.3333, 81.082) (-117.937, 0.3333, -37.8049) (-117.937, 0.3333, -0.0002) (-78.2536, 1.3333, 41.9552)
move_face "Flächen versetzen3" offset -0.2 5 faces at (-114.4577, 0, 1.8856) (-117.239, 0, 2.7813) (117.239, 0, 2.7813) (114.4577, 0, 1.8856) (39.3659, 0, 78.7688)
extrude "Extrusion10" add sketch "Skizze1" against normal blind 13 contours L120 L121 L122 L123
sketch "Skizze2" plane through (0, 0, 23) normal (0, 0, 1) x (-1, 0, 0)
  line L0 (-55, 3) -> (55, 3)
  line L1 (55, 3) -> (55, 13)
  line L2 (55, 13) -> (-55, 13)
  line L3 (-55, 13) -> (-55, 3)
  line L4 (0, 30) -> (0, -10) construction
  line L5 (-61.8127, 0) -> (75, 0) construction
  line L6 (-64.2642, 8.2) -> (72.144, 8.2) construction
  circle A0 centre (45, 8.2) radius 1.25
  circle A1 centre (0, 8.2) radius 1.25
  circle A2 centre (-45, 8.2) radius 1.25
  line L7 (-43.7298, 6) -> (-42.4597, 8.2)
  line L8 (-42.4597, 8.2) -> (-43.7298, 10.4)
  line L9 (-43.7298, 10.4) -> (-46.2702, 10.4)
  line L10 (-46.2702, 10.4) -> (-47.5403, 8.2)
  line L11 (-47.5403, 8.2) -> (-46.2702, 6)
  line L12 (-46.2702, 6) -> (-43.7298, 6)
  line L13 (1.2702, 6) -> (2.5403, 8.2)
  line L14 (2.5403, 8.2) -> (1.2702, 10.4)
  line L15 (1.2702, 10.4) -> (-1.2702, 10.4)
  line L16 (-1.2702, 10.4) -> (-2.5403, 8.2)
  line L17 (-2.5403, 8.2) -> (-1.2702, 6)
  line L18 (-1.2702, 6) -> (1.2702, 6)
  line L19 (46.2702, 6) -> (47.5403, 8.2)
  line L20 (47.5403, 8.2) -> (46.2702, 10.4)
  line L21 (46.2702, 10.4) -> (43.7298, 10.4)
  line L22 (43.7298, 10.4) -> (42.4597, 8.2)
  line L23 (42.4597, 8.2) -> (43.7298, 6)
  line L24 (43.7298, 6) -> (46.2702, 6)
  line L25 (-47.5403, 8.2) -> (-42.4597, 8.2)
  line L26 (-42.4597, 8.2) -> (-42.4597, 10.4)
  line L27 (-42.4597, 10.4) -> (-47.5403, 10.4)
  line L28 (-47.5403, 10.4) -> (-47.5403, 8.2)
  line L29 (-2.5403, 8.2) -> (2.5403, 8.2)
  line L30 (2.5403, 8.2) -> (2.5403, 10.4)
  line L31 (2.5403, 10.4) -> (-2.5403, 10.4)
  line L32 (-2.5403, 10.4) -> (-2.5403, 8.2)
  line L33 (42.4597, 8.2) -> (47.5403, 8.2)
  line L34 (47.5403, 8.2) -> (47.5403, 10.4)
  line L35 (47.5403, 10.4) -> (42.4597, 10.4)
  line L36 (42.4597, 10.4) -> (42.4597, 8.2)
  point P0 (-45, 8.2)
  point P1 (0, 8.2)
  point P2 (45, 8.2)
  dimension "d118" = 8.2
  dimension "d119" = 45
  dimension "d120" = 45
  dimension "d121" = 2.5
  dimension "d122" = 2.5
  dimension "d123" = 2.5
  dimension "d124" = 4.4
  dimension "d125" = 4.4
  dimension "d126" = 4.4
  constraint vertical L4
  constraint coincident origin L4
  constraint horizontal L5
  constraint perpendicular L1 L6
  constraint coincident origin L5
  constraint coincident L6 P2
  constraint coincident L6 P1
  constraint coincident L4 P1
  constraint coincident L6 P0
  constraint coincident P0 A2.centre
  constraint coincident P1 A1.centre
  constraint coincident P2 A0.centre
  constraint horizontal L24
  constraint horizontal L18
  constraint horizontal L12
  constraint horizontal L25
  constraint vertical L26
  constraint horizontal L27
  constraint vertical L28
  constraint horizontal L29
  constraint vertical L30
  constraint horizontal L31
  constraint vertical L32
  constraint horizontal L33
  constraint vertical L34
  constraint horizontal L35
  constraint vertical L36
  constraint coincident L19.end L34
  constraint coincident L20.end L35
  constraint coincident L13.end L14.start
  constraint coincident L14.end L31
  constraint coincident L7.end L8.start
  constraint coincident L8.end L27
  measures "d118" distance of L5 L6
  measures "d119" distance of P1 P0
  measures "d120" distance of P2 P1
  measures "d121" diameter of A0
  measures "d122" diameter of A1
  measures "d123" diameter of A2
  measures "d124" distance of L9 L12
  measures "d125" distance of L15 L18
  measures "d126" distance of L21 L24
extrude "Extrusion11" cut sketch "Skizze2" against normal blind 10 contours A0 L33 | A0 L33 | A1 L29 | A1 L29 | A2 L25 | A2 L25
extrude "Extrusion12" cut sketch "Skizze2" against normal blind 4 contours A0 L19 L23 L24 L33 | A0 L20 L21 L22 L33 L35 | L20 L34 L35 | L22 L35 L36 | A1 L13 L17 L18 L29 | A1 L14 L15 L16 L29 L31 | L14 L30 L31 | L16 L31 L32 | A2 L7 L11 L12 L25 | A2 L8 L9 L10 L25 L27 | L8 L26 L27 | L10 L27 L28
extrude "Extrusion13" add sketch "Skizze2" against normal blind 2 contours A0 L19 L23 L24 L33 | A0 L20 L21 L22 L33 L35 | L20 L34 L35 | L22 L35 L36 | A1 L13 L17 L18 L29 | A1 L14 L15 L16 L29 L31 | L14 L30 L31 | L16 L31 L32 | A2 L7 L11 L12 L25 | A2 L8 L9 L10 L25 L27 | L8 L26 L27 | L10 L27 L28
equation "d71 = d70"
equation "d73 = d72"
equation "d75 = d74"
equation "d77 = d76"
equation "d118 = 8 mm + 0.2 mm"
equation "d162 = ( -7.895 * 3 ) * 1 mm"
equation "d169 = 7.895 mm * 2"
named bodies: "back"
